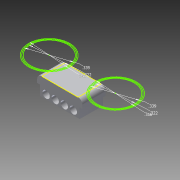
# Autodesk Inventor part: 2mmWireBoardConn_plug
Saved by Autodesk Inventor 2014 (Build 180170000, 170)
## iProperties
Created: 2015-11-06
Part Number: 2mmWireBoardConn_plug
Material: Generic
Document SubType Name: Modeling
Designer: Owner
Density: 1 g/cm^3
Appearance: Smooth - White
Author: Owner
Autodesk Inventor part; units mm, degrees
ref_plane "YZ Plane" through (0, 0, 0) normal (1, 0, 0) x (0, 1, 0)
ref_plane "XZ Plane" through (0, 0, 0) normal (0, 1, 0) x (-1, 0, 0)
ref_plane "XY Plane" through (0, 0, 0) normal (0, 0, 1) x (1, 0, 0)
sketch "Sketch1" plane through (0, 0, 0) normal (0, 0, 1) x (1, 0, 0)
  line L0 (-4.6623, 0.8488) -> (4.1377, 0.8488)
  line L1 (4.1377, 0.8488) -> (4.1377, -2.3302)
  line L2 (4.1377, -2.3302) -> (-4.6623, -2.3302)
  line L3 (-4.6623, -2.3302) -> (-4.6623, 0.8488)
  line L4 (-4.2623, 1.6698) -> (3.7377, 1.6698)
  line L5 (4.7377, 0.6698) -> (4.7377, -0.1302)
  line L6 (4.7377, -0.1302) -> (-5.2623, -0.1302)
  line L7 (-5.2623, -0.1302) -> (-5.2623, 0.6698)
  arc A0 (-4.2623, 1.6698) -> (-5.2623, 0.6698) centre (-4.2623, 0.6698) ccw
  arc A1 (4.7377, 0.6698) -> (3.7377, 1.6698) centre (3.7377, 0.6698) ccw
  circle A2 centre (-3.2623, -1.3302) radius 0.8
  line L8 (-3.2623, -1.3302) -> (2.6542, -1.3302) construction
  circle A3 centre (-1.2623, -1.3302) radius 0.8
  circle A4 centre (0.7377, -1.3302) radius 0.8
  circle A5 centre (2.7377, -1.3302) radius 0.8
  point P0 (0, 0)
  point P1 (-5.2623, 1.6698)
  point P2 (4.7377, 1.6698)
  dimension "d0" = 10
  dimension "d1" = 4
  dimension "d2" = 8.8
  dimension "d3" = 0.6
  dimension "d4" = 1.8
  dimension "d7" = 1
  dimension "d8" = 1
  dimension "d9" = 1.6
  dimension "d10" = 1.6
  dimension "d11" = 1.6
  dimension "d12" = 1.6
  dimension "d13" = 2
  dimension "d14" = 2
  dimension "d15" = 2
  dimension "d16" = 2
  constraints: 18 end point, 7 point on line, 6 centre point, 4 parallel, 4 point on circle, 4 tangent, 3 perpendicular, 2 horizontal, 1 equal radius
  measures "d0" distance of point (-5.262, 1.67) point (4.738, 1.67)
  measures "d1" distance between parallel lines of L2 L4
  measures "d2" distance of L1.end L2.end
  measures "d3" distance between parallel lines of L7 L3
  measures "d4" distance of L6.end point (-5.262, 1.67)
  measures "d7" radius of A0
  measures "d8" distance between parallel lines of L2 L8
  measures "d9" diameter of A2
  measures "d10" diameter of A3
  measures "d11" diameter of A4
  measures "d12" diameter of A5
  measures "d13" distance from line of L7 L8.start
  measures "d14" distance of A3.centre L8.start
  measures "d15" distance of A4.centre A3.centre
  measures "d16" distance of A5.centre A4.centre
extrude "Extrusion1" add sketch "Sketch1" along normal blind 5.1
sketch "Sketch3" plane through (-4.2623, 1.6698, 0) normal (0, 1, 0) x (1, 0, 0)
  line L0 (8, 0) -> (0, 0) projected
  line L1 (0, 0) -> (0, -5.1) projected
  line L2 (8, -5.1) -> (0, -5.1) projected
  line L3 (8, 0) -> (8, -5.1) projected
  circle A0 centre (11.8741, -0.2668) radius 4.9
  circle A1 centre (11.8741, -0.2668) radius 5.145
  circle A2 centre (11.8741, -0.2668) radius 4.655
  circle A3 centre (-3.7362, 0) radius 4.9
  circle A4 centre (-3.7362, 0) radius 5.145
  circle A5 centre (-3.7362, 0) radius 4.655
  point P0 (4.2623, 0)
  dimension "d17" = 9.8
  dimension "d18" = 9.31
  dimension "d19" = 10.29
  dimension "d23" = 9.8
  dimension "d24" = 9.31
  dimension "d25" = 10.29
  constraints: 6 centre point, 4 coincident
  measures "d17" diameter of A0
  measures "d18" diameter of A2
  measures "d19" diameter of A1
  measures "d23" diameter of A3
  measures "d24" diameter of A5
  measures "d25" diameter of A4
body "Solid1"
